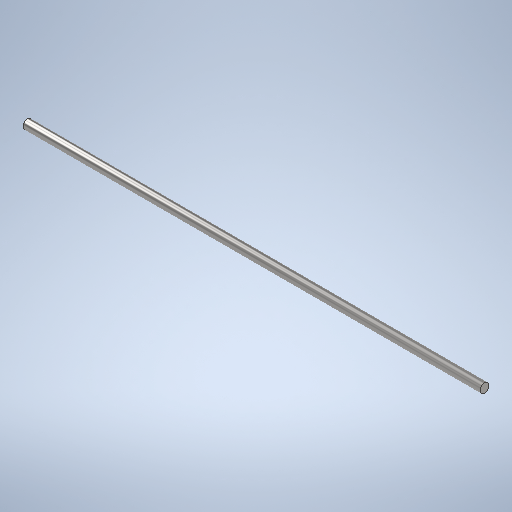
# Autodesk Inventor part: shaft
Saved by Autodesk Inventor 2026.1 (Build 301233020, 233B)
## iProperties
Created: 2026-01-22
Part Number: shaft
Material: Steel, Alloy
Document SubType Name: Modeling
Designer: user
Density: 7.73 g/cm^3
Appearance: Semi-Polished
Mass: 155.421 g
Surface Area: 101.536 cm^2
Volume: 20.1062 cm^3
Author: user
Autodesk Inventor part; units mm, degrees
ref_plane "YZ Plane" through (0, 0, 0) normal (1, 0, 0) x (0, 1, 0)
sketch "Sketch1" plane through (0, 0, 0) normal (1, 0, 0) x (0, 1, 0)
  circle A0 centre (0, 0) radius 4
  dimension "d0" = 8
  constraints: 1 centre point, 1 coincident
  measures "d0" diameter of A0
extrude "Extrusion1" add sketch "Sketch1" along normal blind 400
ref_plane "Work Plane1" through (0, 0, 0) normal (-1, 0, 0) x (0, 0, 1)
ref_plane "Work Plane2" through (400, 0, 0) normal (1, 0, 0) x (0, 0, -1)
body "Solid1"
